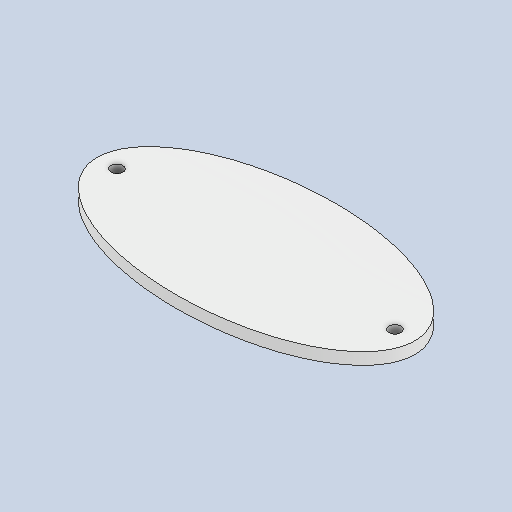
# Autodesk Inventor part: Forearm_4
Saved by Autodesk Inventor 2022 (Build 260153000, 153)
## iProperties
Created: 2023-01-17
Part Number: Forearm_4
Material: ABS Plastic
Document SubType Name: Modeling
Designer: 48735
Density: 1.06 g/cm^3
Appearance: Smooth - White
Author: 48735
Autodesk Inventor part; units mm, degrees
ref_plane "YZ Plane" through (0, 0, 0) normal (1, 0, 0) x (0, 1, 0)
ref_plane "XZ Plane" through (0, 0, 0) normal (0, 1, 0) x (-1, 0, 0)
ref_plane "XY Plane" through (0, 0, 0) normal (0, 0, 1) x (1, 0, 0)
sketch "Sketch1" plane through (0, 0, 0) normal (0, 1, 0) x (-1, 0, 0)
  ellipse E0 centre (0, 0) end of major axis (-40, 0) minor radius 20
  circle A0 centre (35, 0) radius 1.5
  circle A1 centre (-35, 0) radius 1.5
  constraints: 2 centre point, 1 coincident, 2 other
extrude "Extrusion1" add sketch "Sketch1" along normal blind 3
body "Solid1"
